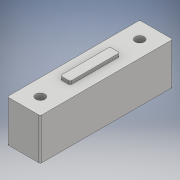
# Autodesk Inventor part: モータースペーサ
Saved by Autodesk Inventor 2017 (Build 210142000, 142)
## iProperties
Part Number: モータースペーサ
Material: 一般
Document SubType Name: Modeling
Designer: highs
Density: 1 g/cm^3
Appearance: 既定
Author: highs
## iProperties of the stored document モータースペーサ_3D プリント.ipt
Part Number: モータースペーサ_3D プリント
Material: 一般
Document SubType Name: Modeling
Designer: highs
Density: 1 g/cm^3
Appearance: 既定
Author: highs
Autodesk Inventor part; units mm, degrees
ref_plane "YZ Plane" through (0, 0, 0) normal (1, 0, 0) x (0, 1, 0)
ref_plane "XZ Plane" through (0, 0, 0) normal (0, 1, 0) x (-1, 0, 0)
ref_plane "XY Plane" through (0, 0, 0) normal (0, 0, 1) x (1, 0, 0)
sketch "スケッチ2" plane through (0, 0, 0) normal (0, 0, 1) x (1, 0, 0)
  line L0 (0, 0) -> (20, 0)
  line L1 (20, 0) -> (20, 80)
  line L2 (20, 80) -> (0, 80)
  line L3 (0, 80) -> (0, 0)
  line L4 (10, 80) -> (10, 0) construction
  circle A0 centre (10, 70) radius 2.75
  circle A1 centre (10, 10) radius 2.75
  dimension "d4" = 20
  dimension "d5" = 80
  dimension "d15" = 10
  dimension "d16" = 10
  dimension "d17" = 5.5
  constraints: 10 end point, 2 centre point, 2 horizontal, 2 midpoint, 2 perpendicular, 2 point on line, 1 equal radius
  measures "d4" distance of L0.start L0.end
  measures "d5" distance of L2.end L0.start
  measures "d15" distance from line of L2 A0.centre
  measures "d16" distance from line of L0 A1.centre
  measures "d17" diameter of A0
extrude "押し出し2" add sketch "スケッチ2" along normal blind 25
sketch "スケッチ4" plane through (0, 0, 25) normal (0, 0, 1) x (1, 0, 0)
  line L0 (0, 0) -> (20, 0) construction
  line L1 (10, 0) -> (10, 80) construction
  line L2 (20, 80) -> (0, 80) construction
  line L3 (0, 80) -> (0, 0) construction
  line L4 (0, 40) -> (20, 40) construction
  line L5 (20, 0) -> (20, 80) construction
  line L6 (13, 25) -> (7, 25)
  line L7 (7, 25) -> (7, 55)
  line L8 (7, 55) -> (13, 55)
  line L9 (13, 55) -> (13, 25)
  line L10 (13, 25) -> (7, 55) construction
  line L11 (7, 25) -> (13, 55) construction
  point P0 (10, 40)
  dimension "d18" = 6
  dimension "d19" = 30
  constraints: 16 end point, 7 midpoint, 2 parallel, 1 horizontal, 1 perpendicular
  measures "d18" distance between parallel lines of L9 L7
  measures "d19" distance of L6.end L7.end
extrude "押し出し4" add sketch "スケッチ4" along normal blind 2
fillet "フィレット1" radius 1 8 edges at (13, 25, 26) (13, 55, 26) (7, 55, 26) (7, 25, 26) (0, 0, 12.5) (20, 0, 12.5) (20, 80, 12.5) (0, 80, 12.5)
